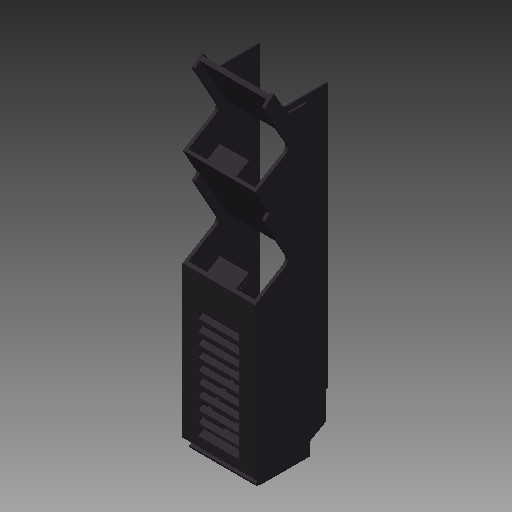
# Autodesk Inventor part: CH20M22 S PPSC BK 2418650000
Saved by Autodesk Inventor 2019.3 (Build 233278000, 278)
## iProperties
Category: PARTsolutions
Company: WEIDMUELLER
Created: 2018-11-15
Part Number: CH20M22 S PPSC BK 2418650000
Material: Generic
Catalog Web Link: www.cadenas.de
Description: CH20M22 S PPSC-CH20M
Vendor: WEIDMUELLER
Document SubType Name: Modeling
Designer: psadmin
Manufacturer: WEIDMUELLER
Mass: 5.52123 g
Surface Area: 130.591 cm^2
Volume: 5.52123 cm^3
Density: 1 g/cm^3
Appearance: PSOLRGB-68-61-68
PSOL_IDENT_0: {$CADENAS_DATA\23d-libs\weidmueller\elektronikgehaeuse\einbaugehaeuse\ch20m\einzelteile\ch20m22-5\ch
PSOL_IDENT_1: 20m22-s-ppsc.prj},204 {VTYP=3D},{NB=CH20M22 S PPSC BK 2418650000},{LINA=CH20M22 S PPSC BK 2418650000
PSOL_IDENT_2: },{NN=CH20M22 S PPSC},{DATE=31.03.2017 09:22:38},{GEOMDATE=18.01.2013 15:12:00},{VERSION=},{LINEID=1
PSOL_IDENT_3: 0},{WBVAR=},{WBNUMERIC=}  {NB=CH20M22 S PPSC BK 2418650000},{LINA=CH20M22 S PPSC BK 2418650000},{KT=
PSOL_IDENT_4: DUMMY},{BEST=2418650000},{BZ=CH20M22 S PPSC BK},{F=schwarz},{FCODE=0.27,0.24,0.27,0.00}
NN: CH20M22 S PPSC
NT: CH20M
NB: CH20M22 S PPSC BK 2418650000
NBSYN: $BZ. $BEST.
LINA: CH20M22 S PPSC BK 2418650000
BEST: 2418650000
BZ: CH20M22 S PPSC BK
F: black
SUPPLIER: WEIDMUELLER
ARTICLENO: CH20M22 S PPSC BK 2418650000
BOMINFO: CH20M22 S PPSC BK 2418650000
CREATOR: CADENAS GmbH
Title: CH20M22 S PPSC BK 2418650000
Author: Cadenas PARTsolutions
Comments: CH20M
Autodesk Inventor part; units mm, degrees
sketch "Sketch_1" plane through (-11.25, 0, 0) normal (1, 0, 0) x (0, 0, -1)
  line L0 (-23.0103, 50.048) -> (-23.0103, 3.2887)
  line L1 (-23.0103, 3.2887) -> (-22.0733, 3.8134)
  line L2 (-22.0733, 3.8134) -> (-21.2148, 1.4617)
  line L3 (-21.2148, 1.4617) -> (-21.9165, 1.1337)
  line L4 (-21.9165, 1.1337) -> (-21.9199, 0.9366)
  arc A0 (-21.9199, 0.9366) -> (-21.0008, 0.2762) centre (-21.2317, 0.9247) ccw
  line L5 (-21.0008, 0.2762) -> (-20.8072, 0.3452)
  line L6 (-20.8072, 0.3452) -> (-20.7292, 0.1315)
  arc A1 (-20.7292, 0.1315) -> (-20.5413, 0) centre (-20.5413, 0.2001) ccw
  line L7 (-20.5413, 0) -> (-4.0008, 0)
  line L8 (-4.0008, 0) -> (-4.0008, 4.6661)
  line L9 (-4.0008, 4.6661) -> (0, 6.9063)
  line L10 (0, 6.9063) -> (0, 97.9887)
  line L11 (0, 97.9887) -> (-12.7393, 97.9887)
  arc A2 (-14.4841, 99.0114) -> (-12.7393, 97.9887) centre (-12.7393, 99.9883) ccw
  line L12 (-14.4841, 99.0114) -> (-16.9901, 103.4868)
  arc A3 (-16.9901, 103.4868) -> (-17.4387, 103.5749) centre (-17.2518, 103.3402) ccw
  arc A4 (-17.4387, 103.5749) -> (-19.8079, 101.4349) centre (-1.3603, 83.3925) ccw
  arc A5 (-19.8079, 101.4349) -> (-19.9262, 100.5441) centre (-19.2718, 100.9105) ccw
  line L13 (-19.9262, 100.5441) -> (-12.9626, 88.1078)
  arc A6 (-13.5948, 85.7488) -> (-12.9626, 88.1078) centre (-14.4895, 87.2528) ccw
  line L14 (-13.5948, 85.7488) -> (-22.7724, 80.2895)
  arc A7 (-22.7724, 80.2895) -> (-22.8446, 80.0198) centre (-22.6701, 80.1176) ccw
  line L15 (-22.8446, 80.0198) -> (-18.5546, 72.3606)
  arc A8 (-18.5546, 72.3606) -> (-19.7416, 71.2061) centre (-1.1704, 53.2996) ccw
  arc A9 (-19.7416, 71.2061) -> (-19.8561, 70.319) centre (-19.2016, 70.6855) ccw
  line L16 (-19.8561, 70.319) -> (-12.9626, 58.0078)
  arc A10 (-13.5948, 55.6488) -> (-12.9626, 58.0078) centre (-14.4895, 57.1528) ccw
  line L17 (-13.5948, 55.6488) -> (-23.0103, 50.048)
  constraints: 36 end point, 22 point on circle, 11 centre point
extrude "Extrusion1" add sketch "Sketch_1" along normal blind 0.95
sketch "Sketch_3" plane through (-10.3, 0, 0) normal (1, 0, 0) x (0, 0, -1)
  line L0 (-23.0103, 49.9343) -> (-23.0103, 3.2887)
  line L1 (-23.0103, 3.2887) -> (-22.0733, 3.8134)
  line L2 (-22.0733, 3.8134) -> (-21.2148, 1.4617)
  line L3 (-21.2148, 1.4617) -> (-21.9165, 1.1337)
  line L4 (-21.9165, 1.1337) -> (-21.9199, 0.9366)
  arc A0 (-21.9199, 0.9366) -> (-21.0008, 0.2762) centre (-21.2317, 0.9247) ccw
  line L5 (-21.0008, 0.2762) -> (-20.8072, 0.3452)
  line L6 (-20.8072, 0.3452) -> (-20.7292, 0.1315)
  arc A1 (-20.7292, 0.1315) -> (-20.5413, 0) centre (-20.5413, 0.2001) ccw
  line L7 (-20.5413, 0) -> (-4.3753, 0)
  arc A2 (-4.3753, 0) -> (-4.1753, 0.2) centre (-4.3753, 0.2) ccw
  line L8 (-4.1753, 0.2) -> (-4.1753, 1)
  line L9 (-4.1753, 1) -> (-20.1942, 1)
  line L10 (-20.1942, 1) -> (-21.7598, 5.2887)
  line L11 (-21.7598, 5.2887) -> (-21.7598, 6.3887)
  line L12 (-21.7598, 6.3887) -> (-21.1202, 6.7468)
  line L13 (-21.1202, 6.7468) -> (-21.7598, 7.8887)
  line L14 (-21.7598, 7.8887) -> (-21.7598, 49.3377)
  line L15 (-21.7598, 49.3377) -> (-17.5997, 51.8124)
  line L16 (-17.5997, 51.8124) -> (-18.2106, 52.9031)
  line L17 (-18.2106, 52.9031) -> (-22.9125, 50.1062)
  arc A3 (-22.9125, 50.1062) -> (-23.0103, 49.9343) centre (-22.8103, 49.9343) ccw
  constraints: 36 end point, 8 point on circle, 4 centre point
extrude "Extrusion2" add sketch "Sketch_3" along normal blind 20.6
sketch "Sketch_4" plane through (11.25, 0, 0) normal (1, 0, 0) x (0, 0, -1)
  line L0 (-23.0103, 50.048) -> (-23.0103, 3.2887)
  line L1 (-23.0103, 3.2887) -> (-22.0733, 3.8134)
  line L2 (-22.0733, 3.8134) -> (-21.2148, 1.4617)
  line L3 (-21.2148, 1.4617) -> (-21.9165, 1.1337)
  line L4 (-21.9165, 1.1337) -> (-21.9199, 0.9366)
  arc A0 (-21.9199, 0.9366) -> (-21.0008, 0.2762) centre (-21.2317, 0.9247) ccw
  line L5 (-21.0008, 0.2762) -> (-20.8072, 0.3452)
  line L6 (-20.8072, 0.3452) -> (-20.7292, 0.1315)
  arc A1 (-20.7292, 0.1315) -> (-20.5413, 0) centre (-20.5413, 0.2001) ccw
  line L7 (-20.5413, 0) -> (-4.0008, 0)
  line L8 (-4.0008, 0) -> (-4.0008, 4.6661)
  line L9 (-4.0008, 4.6661) -> (0, 6.9063)
  line L10 (0, 6.9063) -> (0, 97.9887)
  line L11 (0, 97.9887) -> (-12.7393, 97.9887)
  arc A2 (-14.4841, 99.0114) -> (-12.7393, 97.9887) centre (-12.7393, 99.9883) ccw
  line L12 (-14.4841, 99.0114) -> (-16.9901, 103.4868)
  arc A3 (-16.9901, 103.4868) -> (-17.4387, 103.5749) centre (-17.2518, 103.3402) ccw
  arc A4 (-17.4387, 103.5749) -> (-19.8079, 101.4349) centre (-1.3603, 83.3925) ccw
  arc A5 (-19.8079, 101.4349) -> (-19.9262, 100.5441) centre (-19.2718, 100.9105) ccw
  line L13 (-19.9262, 100.5441) -> (-12.9626, 88.1078)
  arc A6 (-13.5948, 85.7488) -> (-12.9626, 88.1078) centre (-14.4895, 87.2528) ccw
  line L14 (-13.5948, 85.7488) -> (-22.7724, 80.2895)
  arc A7 (-22.7724, 80.2895) -> (-22.8446, 80.0198) centre (-22.6701, 80.1176) ccw
  line L15 (-22.8446, 80.0198) -> (-18.5546, 72.3606)
  arc A8 (-18.5546, 72.3606) -> (-19.7416, 71.2061) centre (-1.1704, 53.2996) ccw
  arc A9 (-19.7416, 71.2061) -> (-19.8561, 70.319) centre (-19.2016, 70.6855) ccw
  line L16 (-19.8561, 70.319) -> (-12.9626, 58.0078)
  arc A10 (-13.5948, 55.6488) -> (-12.9626, 58.0078) centre (-14.4895, 57.1528) ccw
  line L17 (-13.5948, 55.6488) -> (-23.0103, 50.048)
  constraints: 36 end point, 22 point on circle, 11 centre point
extrude "Extrusion3" add sketch "Sketch_4" against normal blind 0.95
sketch "Sketch_2" plane through (0, 0, 0) normal (1, 0, 0) x (0, 1, 0)
  line L0 (4.1065, 5) -> (0, 5)
  line L1 (0, 5) -> (0, 0)
  line L2 (0, 0) -> (6.9063, 0)
  line L3 (6.9063, 0) -> (4.1065, 5)
  constraints: 8 end point
sketch "Sketch_6" plane through (0, 0, 0) normal (1, 0, 0) x (0, 1, 0)
  arc A0 (80.2895, 22.7721) -> (80.0198, 22.8444) centre (80.1176, 22.6698) ccw
  line L0 (80.0198, 22.8444) -> (57.7128, 10.3499)
  line L1 (57.7128, 10.3499) -> (58.177, 9.5209)
  line L2 (58.177, 9.5209) -> (79.5852, 21.5119)
  line L3 (79.5852, 21.5119) -> (81.9124, 17.5997)
  line L4 (81.9124, 17.5997) -> (83.003, 18.2105)
  line L5 (83.003, 18.2105) -> (80.2895, 22.7721)
  constraints: 12 end point, 2 point on circle, 1 centre point
extrude "Extrusion4" add sketch "Sketch_6" along normal mid plane 20.6
sketch "Sketch_7" plane through (0, 0, 0) normal (1, 0, 0) x (0, 1, 0)
  line L0 (102.5754, 18.6186) -> (87.8128, 10.3499)
  line L1 (87.8128, 10.3499) -> (88.4236, 9.2592)
  line L2 (88.4236, 9.2592) -> (103.4044, 17.6501)
  arc A0 (103.4044, 17.6501) -> (102.5754, 18.6186) centre (83.3925, 1.36) ccw
  constraints: 6 end point, 2 point on circle, 1 centre point
extrude "Extrusion5" add sketch "Sketch_7" along normal mid plane 20.6
sketch "Sketch_10" plane through (4.5, 0, 0) normal (1, 0, 0) x (0, 0, -1)
  line L0 (-22.4896, 81.3307) -> (-8.8659, 57.0076)
  line L1 (-8.8659, 57.0076) -> (-16.3535, 52.5536)
  line L2 (-16.3535, 52.5536) -> (-17.3312, 54.2991)
  line L3 (-17.3312, 54.2991) -> (-22.4896, 51.2307)
  line L4 (-22.4896, 51.2307) -> (-8.8659, 26.9076)
  line L5 (-8.8659, 26.9076) -> (0, 26.9076)
  line L6 (0, 26.9076) -> (0, 92.3815)
  line L7 (0, 92.3815) -> (-16.3535, 82.6536)
  line L8 (-16.3535, 82.6536) -> (-17.3312, 84.3992)
  line L9 (-17.3312, 84.3992) -> (-22.4896, 81.3307)
  constraints: 20 end point
extrude "Extrusion6" cut sketch "Sketch_10" along normal blind 5.8
sketch "Sketch_11" plane through (-4.5, 0, 0) normal (1, 0, 0) x (0, 0, -1)
  line L0 (-22.4896, 81.3307) -> (-8.8659, 57.0076)
  line L1 (-8.8659, 57.0076) -> (-16.3535, 52.5536)
  line L2 (-16.3535, 52.5536) -> (-17.3312, 54.2991)
  line L3 (-17.3312, 54.2991) -> (-22.4896, 51.2307)
  line L4 (-22.4896, 51.2307) -> (-8.8659, 26.9076)
  line L5 (-8.8659, 26.9076) -> (0, 26.9076)
  line L6 (0, 26.9076) -> (0, 92.3815)
  line L7 (0, 92.3815) -> (-16.3535, 82.6536)
  line L8 (-16.3535, 82.6536) -> (-17.3312, 84.3992)
  line L9 (-17.3312, 84.3992) -> (-22.4896, 81.3307)
  constraints: 20 end point
extrude "Extrusion7" cut sketch "Sketch_11" against normal blind 5.8
sketch "Sketch_8" plane through (-10.3, 0, 0) normal (1, 0, 0) x (0, 0, -1)
  line L0 (-22.4623, 4.8791) -> (-21.2148, 1.4617)
  line L1 (-21.2148, 1.4617) -> (-21.9165, 1.1337)
  line L2 (-21.9165, 1.1337) -> (-21.9199, 0.9366)
  arc A0 (-21.9199, 0.9366) -> (-21.0008, 0.2762) centre (-21.2317, 0.9247) ccw
  line L3 (-21.0008, 0.2762) -> (-20.8072, 0.3452)
  line L4 (-20.8072, 0.3452) -> (-20.7292, 0.1315)
  arc A1 (-20.7292, 0.1315) -> (-20.5413, 0) centre (-20.5413, 0.2001) ccw
  line L5 (-20.5413, 0) -> (-4.0008, 0)
  line L6 (-4.0008, 0) -> (-4.0008, 4.6661)
  line L7 (-4.0008, 4.6661) -> (0, 6.9063)
  line L8 (0, 6.9063) -> (0, 17.4567)
  line L9 (0, 17.4567) -> (-22.4623, 4.8791)
  constraints: 20 end point, 4 point on circle, 2 centre point
extrude "Extrusion8" add sketch "Sketch_8" along normal blind 1
sketch "Sketch_9" plane through (10.3, 0, 0) normal (1, 0, 0) x (0, 0, -1)
  line L0 (-22.4623, 4.8791) -> (-21.2148, 1.4617)
  line L1 (-21.2148, 1.4617) -> (-21.9165, 1.1337)
  line L2 (-21.9165, 1.1337) -> (-21.9199, 0.9366)
  arc A0 (-21.9199, 0.9366) -> (-21.0008, 0.2762) centre (-21.2317, 0.9247) ccw
  line L3 (-21.0008, 0.2762) -> (-20.8072, 0.3452)
  line L4 (-20.8072, 0.3452) -> (-20.7292, 0.1315)
  arc A1 (-20.7292, 0.1315) -> (-20.5413, 0) centre (-20.5413, 0.2001) ccw
  line L5 (-20.5413, 0) -> (-4.0008, 0)
  line L6 (-4.0008, 0) -> (-4.0008, 4.6661)
  line L7 (-4.0008, 4.6661) -> (0, 6.9063)
  line L8 (0, 6.9063) -> (0, 17.4567)
  line L9 (0, 17.4567) -> (-22.4623, 4.8791)
  constraints: 20 end point, 4 point on circle, 2 centre point
extrude "Extrusion9" add sketch "Sketch_9" against normal blind 1
extrude "Extrusion10" cut sketch "Sketch_2" along normal mid plane 24
sketch "Sketch_14" plane through (-11.25, 0, 0) normal (1, 0, 0) x (0, 0, -1)
  line L0 (-22.0733, 3.8134) -> (-21.2148, 1.4617)
  line L1 (-21.2148, 1.4617) -> (-21.9165, 1.1337)
  line L2 (-21.9165, 1.1337) -> (-21.9199, 0.9366)
  arc A0 (-21.9199, 0.9366) -> (-21.0008, 0.2762) centre (-21.2317, 0.9247) ccw
  line L3 (-21.0008, 0.2762) -> (-20.8072, 0.3452)
  line L4 (-20.8072, 0.3452) -> (-20.7292, 0.1315)
  arc A1 (-20.7292, 0.1315) -> (-20.5413, 0) centre (-20.5413, 0.2001) ccw
  line L5 (-20.5413, 0) -> (-4.0008, 0)
  line L6 (-4.0008, 0) -> (-4.0008, 4.6661)
  line L7 (-4.0008, 4.6661) -> (0, 6.9063)
  line L8 (0, 6.9063) -> (0, 16.173)
  line L9 (0, 16.173) -> (-22.0733, 3.8134)
  constraints: 20 end point, 4 point on circle, 2 centre point
extrude "Extrusion11" cut sketch "Sketch_14" along normal blind 1
sketch "Sketch_15" plane through (11.25, 0, 0) normal (1, 0, 0) x (0, 0, -1)
  line L0 (-22.0733, 3.8134) -> (-21.2148, 1.4617)
  line L1 (-21.2148, 1.4617) -> (-21.9165, 1.1337)
  line L2 (-21.9165, 1.1337) -> (-21.9199, 0.9366)
  arc A0 (-21.9199, 0.9366) -> (-21.0008, 0.2762) centre (-21.2317, 0.9247) ccw
  line L3 (-21.0008, 0.2762) -> (-20.8072, 0.3452)
  line L4 (-20.8072, 0.3452) -> (-20.7292, 0.1315)
  arc A1 (-20.7292, 0.1315) -> (-20.5413, 0) centre (-20.5413, 0.2001) ccw
  line L5 (-20.5413, 0) -> (-4.0008, 0)
  line L6 (-4.0008, 0) -> (-4.0008, 4.6661)
  line L7 (-4.0008, 4.6661) -> (0, 6.9063)
  line L8 (0, 6.9063) -> (0, 16.173)
  line L9 (0, 16.173) -> (-22.0733, 3.8134)
  constraints: 20 end point, 4 point on circle, 2 centre point
extrude "Extrusion12" cut sketch "Sketch_15" against normal blind 1
sketch "Sketch_16" plane through (-11.25, 0, 0) normal (1, 0, 0) x (0, 0, -1)
  line L0 (-15.1473, 100.2) -> (-13.48, 97.2228)
  arc A0 (-13.48, 97.2228) -> (-11.735, 96.2) centre (-11.735, 98.2) ccw
  line L1 (-11.735, 96.2) -> (-7, 96.2)
  line L2 (-7, 96.2) -> (-7, 0)
  line L3 (-7, 0) -> (1, 0)
  line L4 (1, 0) -> (1, 100.2)
  line L5 (1, 100.2) -> (-15.1473, 100.2)
  constraints: 12 end point, 2 point on circle, 1 centre point
extrude "Extrusion13" cut sketch "Sketch_16" along normal blind 0.5
sketch "Sketch_17" plane through (11.25, 0, 0) normal (1, 0, 0) x (0, 0, -1)
  line L0 (-15.1473, 100.2) -> (-13.48, 97.2228)
  arc A0 (-13.48, 97.2228) -> (-11.735, 96.2) centre (-11.735, 98.2) ccw
  line L1 (-11.735, 96.2) -> (-7, 96.2)
  line L2 (-7, 96.2) -> (-7, 0)
  line L3 (-7, 0) -> (1, 0)
  line L4 (1, 0) -> (1, 100.2)
  line L5 (1, 100.2) -> (-15.1473, 100.2)
  constraints: 12 end point, 2 point on circle, 1 centre point
extrude "Extrusion14" cut sketch "Sketch_17" against normal blind 0.5
sketch "Sketch_19" plane through (-4.5, 0, 0) normal (1, 0, 0) x (0, 0, -1)
  line L0 (-22.1228, 80.6758) -> (-18.5542, 74.3046)
  line L1 (-18.5542, 74.3046) -> (-14.6419, 76.6318)
  line L2 (-14.6419, 76.6318) -> (-18.2105, 83.003)
  line L3 (-18.2105, 83.003) -> (-22.1228, 80.6758)
  constraints: 8 end point
extrude "Extrusion15" add sketch "Sketch_19" along normal blind 0.9
sketch "Sketch_20" plane through (4.5, 0, 0) normal (1, 0, 0) x (0, 0, -1)
  line L0 (-22.1228, 80.6758) -> (-18.5542, 74.3046)
  line L1 (-18.5542, 74.3046) -> (-14.6419, 76.6318)
  line L2 (-14.6419, 76.6318) -> (-18.2105, 83.003)
  line L3 (-18.2105, 83.003) -> (-22.1228, 80.6758)
  constraints: 8 end point
extrude "Extrusion16" add sketch "Sketch_20" against normal blind 0.9
sketch "Sketch_21" plane through (-4.5, 0, 0) normal (1, 0, 0) x (0, 0, -1)
  line L0 (-21.8, 49.3134) -> (-21.8, 42.2739)
  line L1 (-21.8, 42.2739) -> (-14.642, 46.5318)
  line L2 (-14.642, 46.5318) -> (-17.5995, 51.812)
  line L3 (-17.5995, 51.812) -> (-21.8, 49.3134)
  constraints: 8 end point
extrude "Extrusion17" add sketch "Sketch_21" along normal blind 0.9
sketch "Sketch_22" plane through (4.5, 0, 0) normal (1, 0, 0) x (0, 0, -1)
  line L0 (-21.8, 49.3134) -> (-21.8, 42.2739)
  line L1 (-21.8, 42.2739) -> (-14.642, 46.5318)
  line L2 (-14.642, 46.5318) -> (-17.5995, 51.812)
  line L3 (-17.5995, 51.812) -> (-21.8, 49.3134)
  constraints: 8 end point
extrude "Extrusion18" add sketch "Sketch_22" against normal blind 0.9
sketch "Sketch_5" plane through (0, 0, 0) normal (1, 0, 0) x (0, 1, 0)
  line L0 (4.9971, 24.7) -> (8.5307, 19.7)
  line L1 (8.5307, 19.7) -> (41.25, 19.7)
  line L2 (41.25, 19.7) -> (41.25, 21.7)
  line L3 (41.25, 21.7) -> (39.1298, 24.7)
  line L4 (39.1298, 24.7) -> (36.4971, 24.7)
  line L5 (36.4971, 24.7) -> (38.6173, 21.7)
  line L6 (38.6173, 21.7) -> (37.75, 21.7)
  line L7 (37.75, 21.7) -> (35.6298, 24.7)
  line L8 (35.6298, 24.7) -> (32.9971, 24.7)
  line L9 (32.9971, 24.7) -> (35.1173, 21.7)
  line L10 (35.1173, 21.7) -> (34.25, 21.7)
  line L11 (34.25, 21.7) -> (32.1298, 24.7)
  line L12 (32.1298, 24.7) -> (29.4971, 24.7)
  line L13 (29.4971, 24.7) -> (31.6173, 21.7)
  line L14 (31.6173, 21.7) -> (30.75, 21.7)
  line L15 (30.75, 21.7) -> (28.6298, 24.7)
  line L16 (28.6298, 24.7) -> (25.9971, 24.7)
  line L17 (25.9971, 24.7) -> (28.1173, 21.7)
  line L18 (28.1173, 21.7) -> (27.25, 21.7)
  line L19 (27.25, 21.7) -> (25.1298, 24.7)
  line L20 (25.1298, 24.7) -> (22.4971, 24.7)
  line L21 (22.4971, 24.7) -> (24.6173, 21.7)
  line L22 (24.6173, 21.7) -> (23.75, 21.7)
  line L23 (23.75, 21.7) -> (21.6298, 24.7)
  line L24 (21.6298, 24.7) -> (18.9971, 24.7)
  line L25 (18.9971, 24.7) -> (21.1173, 21.7)
  line L26 (21.1173, 21.7) -> (20.25, 21.7)
  line L27 (20.25, 21.7) -> (18.1298, 24.7)
  line L28 (18.1298, 24.7) -> (15.4971, 24.7)
  line L29 (15.4971, 24.7) -> (17.6173, 21.7)
  line L30 (17.6173, 21.7) -> (16.75, 21.7)
  line L31 (16.75, 21.7) -> (14.6298, 24.7)
  line L32 (14.6298, 24.7) -> (11.9971, 24.7)
  line L33 (11.9971, 24.7) -> (14.1173, 21.7)
  line L34 (14.1173, 21.7) -> (13.25, 21.7)
  line L35 (13.25, 21.7) -> (11.1298, 24.7)
  line L36 (11.1298, 24.7) -> (8.4971, 24.7)
  line L37 (8.4971, 24.7) -> (10.6173, 21.7)
  line L38 (10.6173, 21.7) -> (9.75, 21.7)
  line L39 (9.75, 21.7) -> (7.6298, 24.7)
  line L40 (7.6298, 24.7) -> (4.9971, 24.7)
  constraints: 82 end point
extrude "Extrusion19" cut sketch "Sketch_5" along normal mid plane 12.5
ref_plane "mitBase_XY" through (0, 0, -29.84) normal (0, 0, 1) x (1, 0, 0)
ref_plane "mitBase_YZ" through (0, 0, -29.84) normal (1, 0, 0) x (0, 1, 0)
ref_plane "mitBase_ZX" through (0, 0, -29.84) normal (0, 1, 0) x (0, 0, 1)
body "Solid1"
